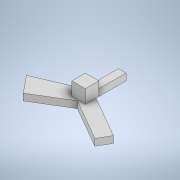
# Autodesk Inventor part: testPart
Saved by Autodesk Inventor 2021.1 (Build 251245010, 245A)
## iProperties
Created: 2020-10-05
Part Number: testPart
Material: Generic
Document SubType Name: Modeling
Designer: robst
Density: 1 g/cm^3
Appearance: Default
Author: robst
Autodesk Inventor part; units mm, degrees
ref_plane "XZ Plane" through (0, 0, 0) normal (0, 1, 0) x (-1, 0, 0)
ref_plane "XY Plane" through (0, 0, 0) normal (0, 0, 1) x (1, 0, 0)
sketch "Sketch2" plane through (0, 0, 0) normal (0, 1, 0) x (-1, 0, 0)
  line L0 (-12.7, 12.7) -> (-12.7, -12.7)
  line L1 (-12.7, -12.7) -> (12.7, -12.7)
  line L2 (12.7, -12.7) -> (12.7, 12.7)
  line L3 (12.7, 12.7) -> (-12.7, 12.7)
  line L4 (-12.7, 12.7) -> (12.7, -12.7) construction
  line L5 (-12.7, -12.7) -> (12.7, 12.7) construction
  point P0 (0, 0)
  dimension "d0" = 25.4
  dimension "d1" = 25.4
  constraints: 12 end point, 2 midpoint, 2 parallel, 1 perpendicular, 1 vertical
  measures "d0" distance of L0.start L0.end
  measures "d1" distance of L1.end L0.end
extrude "Extrusion1" add sketch "Sketch2" along normal blind 25.4
sketch "Sketch9" plane through (0, 0, 0) normal (0, -1, 0) x (1, 0, 0)
  line L0 (0, 0) -> (0, -76.2)
  line L1 (0, 0) -> (0, -42.3666) construction
  line L2 (0, 0) -> (83.3296, 48.1103) construction
  line L3 (0, 0) -> (-72.4381, 41.8221) construction
  line L4 (83.3296, 48.1103) -> (89.6796, 37.1118)
  line L5 (89.6796, 37.1118) -> (6.35, -10.9985)
  line L6 (6.35, -10.9985) -> (0, 0)
  line L7 (0, 0) -> (-6.35, 10.9985)
  line L8 (-6.35, 10.9985) -> (76.9796, 59.1089)
  line L9 (76.9796, 59.1089) -> (83.3296, 48.1103)
  line L10 (-72.4381, 41.8221) -> (-63.7028, 52.6015)
  line L11 (-63.7028, 52.6015) -> (7.6709, 9.4659)
  line L12 (7.6709, 9.4659) -> (0, 0)
  line L13 (-19.0415, -9.4974) -> (0, 0)
  line L14 (-19.0415, -9.4974) -> (-89.3838, 20.9111)
  line L15 (-89.3838, 20.9111) -> (-72.4381, 41.8221)
  line L16 (0, -76.2) -> (14.3386, -76.2)
  line L17 (14.3386, -76.2) -> (14.3386, 0)
  line L18 (14.3386, 0) -> (0, 0)
  line L19 (0, 0) -> (-14.3386, 0)
  line L20 (-14.3386, 0) -> (-14.3386, -76.2)
  line L21 (-14.3386, -76.2) -> (0, -76.2)
  point P0 (-0.4762, 14.3898)
  point P1 (-14.3386, -7.1517)
  dimension "d23" = 76.2
  dimension "d24" = 0
  dimension "d25" = 120
  dimension "d26" = 120
  dimension "d27" = 25.4
  constraints: 44 end point, 8 parallel, 6 collinear, 1 horizontal, 1 perpendicular, 1 point on line, 1 vertical
  measures "d23" distance of L0.start L0.end
  measures "d24" distance between parallel lines of L0 L1
  measures "d25" angle of L2 L0
  measures "d26" angle of L3 L0
  measures "d27" distance between parallel lines of L5 L8
extrude "Extrusion8" add sketch "Sketch9" along normal blind 12.7 contours L18 L17 L5 L6 | L19 L20 L13 L14 L15 L10 L11 L8 L7 | L7 L8 L11 L12 | L0 L21 L20 L13 | L12 L11 L8 L9 L4 L5 L17 L18
sketch "Sketch3" plane through (0, 0, 0) normal (1, 0, 0) x (0, 1, 0)
  line L0 (0, -12.7) -> (0, 12.7) projected
  line L1 (-12.7, 12.7) -> (-12.7, -12.7)
  line L2 (-12.7, -12.7) -> (12.7, -12.7)
  line L3 (12.7, -12.7) -> (12.7, 12.7)
  line L4 (12.7, 12.7) -> (-12.7, 12.7)
  line L5 (-12.7, 12.7) -> (12.7, -12.7) construction
  line L6 (-12.7, -12.7) -> (12.7, 12.7) construction
  point P0 (0, 0)
  dimension "d4" = 25.4
  constraints: 12 end point, 3 parallel, 2 midpoint, 1 perpendicular
  measures "d4" distance of L2.end L1.end
sketch "Sketch4" plane through (0, 0, 0) normal (0, 0, 1) x (1, 0, 0)
  line L0 (-12.7, 12.7) -> (-12.7, 25.4) projected
  line L1 (-38.1, 12.7) -> (-12.7, 12.7) projected
  line L2 (-38.1, -12.7) -> (38.1, -12.7) projected
  line L3 (-12.7, 12.7) -> (12.7, 12.7)
  line L4 (12.7, 12.7) -> (12.7, -12.7)
  line L5 (12.7, -12.7) -> (-12.7, -12.7)
  line L6 (-12.7, -12.7) -> (-12.7, 12.7)
  point P0 (0, 0)
  dimension "d7" = 25.4
  constraints: 8 end point, 2 parallel, 1 horizontal, 1 perpendicular, 1 point on line
  measures "d7" distance of L4.end L5.end
sketch "Sketch5" plane through (0, 25.4, 0) normal (0, 1, 0) x (1, 0, 0)
  line L0 (-5.1393, -5.5117) -> (5.1393, -5.5117)
  line L1 (5.1393, -5.5117) -> (5.1393, 5.5117)
  line L2 (5.1393, 5.5117) -> (-5.1393, 5.5117)
  line L3 (-5.1393, 5.5117) -> (-5.1393, -5.5117)
  line L4 (-5.1393, -5.5117) -> (5.1393, 5.5117) construction
  line L5 (5.1393, -5.5117) -> (-5.1393, 5.5117) construction
  point P0 (0, 0)
  constraints: 12 end point, 2 midpoint, 2 parallel, 1 horizontal, 1 perpendicular
sketch "Sketch6" plane through (0, 0, 0) normal (1, 0, 0) x (0, 1, 0)
  line L0 (-12.7, -12.7) -> (-12.7, 12.7) projected
  line L1 (12.7, 6.35) -> (12.7, -6.35)
  line L2 (12.7, -6.35) -> (-12.7, -6.35)
  line L3 (-12.7, -6.35) -> (-12.7, 6.35)
  line L4 (-12.7, 6.35) -> (12.7, 6.35)
  line L5 (12.7, 6.35) -> (-12.7, -6.35) construction
  line L6 (12.7, -6.35) -> (-12.7, 6.35) construction
  point P0 (0, 0)
  dimension "d12" = 12.7
  constraints: 12 end point, 2 midpoint, 2 parallel, 1 perpendicular, 1 vertical
  measures "d12" distance of L1.start L1.end
sketch "Sketch7" plane through (5.1393, 25.4, 5.5117) normal (0.5, 0, -0.866) x (0, 1, 0)
  line L0 (-38.279, -18.672) -> (-38.279, 4.2588)
  line L1 (-38.279, 4.2588) -> (-12.521, 4.2588)
  line L2 (-12.521, 4.2588) -> (-12.521, -18.672)
  line L3 (-12.521, -18.672) -> (-38.279, -18.672)
  line L4 (-38.279, -18.672) -> (-12.521, 4.2588) construction
  line L5 (-38.279, 4.2588) -> (-12.521, -18.672) construction
  point P0 (-25.4, -7.2066)
  constraints: 12 end point, 2 midpoint, 2 parallel, 1 perpendicular, 1 vertical
sketch "Sketch8" plane through (5.1393, 25.4, 5.5117) normal (0.5, 0, -0.866) x (0, 1, 0)
  line L0 (-38.1, 0.8449) -> (-12.7, 0.8449)
  line L1 (-12.7, 0.8449) -> (-12.7, -15.2581)
  line L2 (-12.7, -15.2581) -> (-38.1, -15.2581)
  line L3 (-38.1, -15.2581) -> (-38.1, 0.8449)
  line L4 (-38.1, 0.8449) -> (-12.7, -15.2581) construction
  line L5 (-12.7, 0.8449) -> (-38.1, -15.2581) construction
  point P0 (-25.4, -7.2066)
  constraints: 12 end point, 2 midpoint, 2 parallel, 1 horizontal, 1 perpendicular
body "Solid1"
